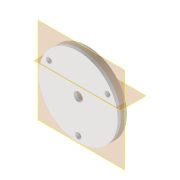
# Autodesk Inventor part: 50_ETL_Top_Seal_v1
Saved by Autodesk Inventor 2022 (Build 260153000, 153)
## iProperties
Created: 2022-01-06
Part Number: 50_ETL_Top_Seal_v1
Material: Generisch
Document SubType Name: Modeling
Designer: diederichbenedict
Density: 1 g/cm^3
Appearance: Vorgabe
Author: diederichbenedict
Autodesk Inventor part; units mm, degrees
ref_plane "YZ Plane" through (0, 0, 0) normal (1, 0, 0) x (0, 1, 0)
ref_plane "XY Plane" through (0, 0, 0) normal (0, 0, 1) x (1, 0, 0)
ref_plane "Arbeitsebene1" through (0, 0, 10) normal (0, 0, 1) x (1, 0, 0)
sketch "Skizze1" plane through (0, 0, 10) normal (0, 0, 1) x (1, 0, 0)
  circle A0 centre (19.3, 0) radius 19.3 projected
  circle A1 centre (5.0106, 8.25) radius 1.4 projected
  circle A2 centre (33.5894, 8.25) radius 1.4 projected
  circle A3 centre (19.3, -16.5) radius 1.5 projected
  circle A4 centre (19.3, 0) radius 2.15
  point P0 (0, 0)
  dimension "d0" = 4.3
  constraints: 1 centre point, 1 coincident, 1 horizontal alignment
  measures "d0" diameter of A4
extrude "Extrusion1" add sketch "Skizze1" along normal blind 1.5
sketch "Skizze2" plane through (19.3, 0, 10) normal (0, 0, -1) x (-1, 0, 0)
  circle A0 centre (0, 0) radius 2.15 projected
  circle A1 centre (0, 0) radius 5.3
  circle A2 centre (0, 0) radius 19.3 projected
  circle A3 centre (0, 0) radius 2.15 projected
  circle A4 centre (0, -16.5) radius 1.5 projected
  circle A5 centre (-14.2894, 8.25) radius 1.4 projected
  circle A6 centre (14.2894, 8.25) radius 1.4 projected
  circle A7 centre (0, 0) radius 5.8
  circle A8 centre (0, 0) radius 8
  circle A9 centre (0, 0) radius 2.65
  point P0 (19.3, 0)
  dimension "d6" = 10.6
  dimension "d7" = 0.5
  dimension "d8" = 16
  dimension "d13" = 0.5
  constraints: 4 centre point, 1 coincident
  measures "d6" diameter of A1
  measures "d7" radial gap between concentric circles of A1 A7
  measures "d8" diameter of A8
  measures "d13" radial gap between concentric circles of A0 A9
extrude "Extrusion2" add sketch "Skizze2" along normal blind 3 contours A2 | A7 | A8 | A9
sketch "Skizze3" plane through (0, 0, 0) normal (0, 1, 0) x (-1, 0, 0)
  point P0 (0, 0)
ref_plane "Arbeitsebene2" through (0, 5, 0) normal (0, 1, 0) x (-1, 0, 0)
